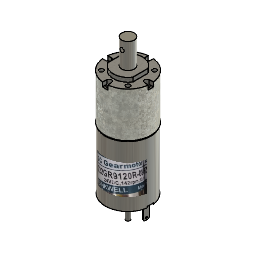
Hennkwell-PZ22GR9120R-084BBH-DC-gearmotor (Autodesk Fusion 360 design; units mm, degrees)
Autodesk Fusion 360 part; units mm, degrees
note: some values were not read from the file. Set by a fixed rule: which sketch regions a step uses.
sketch "Sketch1" plane through (0, 0, 0) normal (0, 1, 0) x (1, 0, 0)
  circle A0 centre (0, 0) radius 11
  circle A1 centre (0, 0) radius 10.8
  dimension "d1" = 22
  dimension "d4" = 21.6
  constraint coincident A0.centre A1.centre
  measures "d1" diameter of A0
  measures "d4" diameter of A1
extrude "Extrude1" add sketch "Sketch1" along normal blind 21.4 contours A0 | A1 makes body 1
extrude "Extrude2" add sketch "Sketch1" against normal blind 29.5 separate body contours A1 makes body 2
sketch "Sketch2" plane through (0, -29.5, 0) normal (0, -1, 0) x (1, 0, 0)
  circle A0 centre (0, 0) radius 10.8
  circle A1 centre (0, 0) radius 3.75
  circle A2 centre (0, 0) radius 1
  dimension "d7" = 7.5
  dimension "d8" = 2
  constraint concentric A0 A1
  constraint coincident A0.centre A1.centre
  measures "d7" diameter of A1
  measures "d8" diameter of A2
extrude "Extrude3" add sketch "Sketch2" along normal blind 2.5 contours A1 | A2 bodies 2
sketch "Sketch3" plane through (0, -29.5, 0) normal (0, -1, 0) x (1, 0, 0)
  circle A0 centre (0, 0) radius 3.75
  circle A1 centre (0, 0) radius 10.8
  line L0 (0, 0) -> (10.8, 0) construction
  line L1 (0, 0) -> (0, 10.8) construction
  line L2 (8.5, -1.5) -> (8.8, -1.5)
  line L3 (8.8, -1.5) -> (8.8, 1.5)
  line L4 (8.8, 1.5) -> (8.5, 1.5)
  line L5 (8.5, 1.5) -> (8.5, -1.5)
  line L6 (8.5, -1.5) -> (8.8, 1.5) construction
  line L7 (8.8, -1.5) -> (8.5, 1.5) construction
  line L8 (-8.8, -1.5) -> (-8.5, 1.5) construction
  line L9 (-8.5, 1.5) -> (-8.5, -1.5)
  line L10 (-8.8, -1.5) -> (-8.8, 1.5)
  line L11 (0, 0) -> (-10.8, 0) construction
  line L12 (-8.5, -1.5) -> (-8.8, 1.5) construction
  line L13 (-8.8, 1.5) -> (-8.5, 1.5)
  line L14 (-8.5, -1.5) -> (-8.8, -1.5)
  line L15 (-8.8, 1.5) -> (-10.6953, 1.5)
  line L16 (-8.8, -1.5) -> (-10.6953, -1.5)
  circle A2 centre (0, 0) radius 10.8
  line L17 (8.8, 1.5) -> (10.6953, 1.5)
  line L18 (8.8, -1.5) -> (10.6953, -1.5)
  point P0 (8.65, 0)
  dimension "d14" = 0.3
  dimension "d15" = 3
  dimension "d16" = 2
  constraint coincident A0.centre A1.centre
  constraint coincident A1 L0.end
  constraint horizontal L0
  constraint coincident A1 L1.end
  constraint perpendicular L0 L1
  constraint horizontal L2
  constraint perpendicular L2 L3
  constraint parallel L2 L4
  constraint parallel L3 L5
  constraint coincident L6 P0
  constraint coincident L7 P0
  constraint coincident L0 P0
  constraint symmetric A0.centre L1 A1.centre
  constraint symmetric L0.end L1 L11.end
  constraint symmetric L1 L2.start L9.end
  constraint symmetric L1 L2.end L8.start
  constraint symmetric L1 L3.end L10.end
  constraint symmetric L1 L4.end L8.end
  constraint coincident A1 L15.end
  constraint perpendicular L10 L15
  constraint coincident A1 L16.end
  constraint perpendicular L10 L16
  constraint coincident A2 L17.end
  constraint perpendicular L3 L17
  constraint coincident A2 L18.end
  constraint perpendicular L3 L18
  measures "d14" distance of L3.end L4.end
  measures "d15" distance of L2.end L3.end
  measures "d16" distance of L0.end L3
extrude "Extrude5" add sketch "Sketch3" along normal blind 6.75 contours L2 L3 L4 L5 | L9 L10 L13 L14 bodies 2
sketch "Sketch4" plane through (-8.8, 0, 0) normal (-1, 0, 0) x (0, 0, 1)
  line L0 (1.5, -29.5) -> (-1.5, -29.5)
  line L1 (-1.5, -29.5) -> (-1.5, -36.25)
  line L2 (-1.5, -36.25) -> (1.5, -36.25)
  line L3 (1.5, -36.25) -> (1.5, -29.5)
  circle A0 centre (0, -35.25) radius 0.5
  dimension "d19" = 1
  dimension "d20" = 1
  dimension "d21" = 1.5
  measures "d19" diameter of A0
  measures "d20" distance of L2 A0.centre
  measures "d21" distance of L1 A0.centre
extrude "Extrude6" cut sketch "Sketch4" against normal blind 1000 contours A0 bodies 2
fillet "Fillet1" radius 1 4 edges at (-8.65, -36.25, -1.5) (-8.65, -36.25, 1.5) (8.65, -36.25, 1.5) (8.65, -36.25, -1.5) on bodies 2
extrude "Extrude7" add sketch "Sketch2" along normal blind 8.4 from surface at 2.5 separate body contours A2 makes body 3
sketch "Sketch5" plane through (0, 21.4, 0) normal (0, 1, 0) x (-1, 0, 0)
  circle A0 centre (0, 0) radius 11
  line L0 (6, -3.625) -> (-6, -3.625)
  line L1 (-6, -3.625) -> (-6, 3.625)
  line L2 (-6, 3.625) -> (6, 3.625)
  line L3 (6, 3.625) -> (6, -3.625)
  line L4 (6, -3.625) -> (-6, 3.625) construction
  line L5 (-6, -3.625) -> (6, 3.625) construction
  line L6 (6, -3.625) -> (6, 3.625)
  arc A1 (-6, -3.6056) -> (6, -3.6056) centre (0, 0) ccw
  arc A2 (6, 3.6056) -> (-6, 3.6056) centre (0, 0) ccw
  circle A3 centre (0, 0) radius 3
  circle A4 centre (0, 0) radius 9
  line L7 (0, 0) -> (0, -11) construction
  line L8 (0, 0) -> (0, 11) construction
  line L9 (0, 0) -> (-11, 0) construction
  line L10 (0, 0) -> (11, 0) construction
  circle A5 centre (9, 0) radius 1.15
  circle A6 centre (0, 9) radius 1.15
  circle A7 centre (-9, 0) radius 1.15
  circle A8 centre (0, -9) radius 1.15
  line L11 (8.9265, -1.1477) -> (10.9258, -1.2756)
  line L12 (8.9265, 1.1477) -> (10.9258, 1.2756)
  line L13 (-8.9265, -1.1477) -> (-10.9258, -1.2756)
  line L14 (-8.9265, 1.1477) -> (-10.9258, 1.2756)
  line L15 (-1.1477, -8.9265) -> (-1.2756, -10.9258)
  line L16 (1.1477, -8.9265) -> (1.2756, -10.9258)
  line L17 (1.1477, 8.9265) -> (1.2756, 10.9258)
  line L18 (-1.1477, 8.9265) -> (-1.2756, 10.9258)
  line L19 (0, 0) -> (-6.3679, 6.36) construction
  circle A9 centre (-6.3679, 6.36) radius 1
  circle A10 centre (6.3679, 6.36) radius 1
  circle A11 centre (-6.3679, -6.36) radius 1
  circle A12 centre (6.3679, -6.36) radius 1
  dimension "d32" = 14
  dimension "d33" = 12
  dimension "d34" = 7.25
  dimension "d37" = 6
  dimension "d40" = 18
  dimension "d41" = 2.3
  dimension "d42" = 2.3
  dimension "d43" = 2.3
  dimension "d44" = 2.3
  dimension "d49" = 2
  constraint coincident A0.centre A1.centre
  constraint horizontal L0
  constraint perpendicular L0 L1
  constraint parallel L0 L2
  constraint parallel L1 L3
  constraint coincident L4 A0.centre
  constraint coincident L5 A0.centre
  constraint coincident L1 A2.end
  constraint coincident L1 A1.start
  constraint coincident L3 A1.end
  constraint coincident L3 A2.start
  constraint concentric A1 A2
  constraint concentric A1 A4
  constraint coincident A0 L7.end
  constraint perpendicular L0 L7
  constraint coincident A0 L8.end
  constraint parallel L7 L8
  constraint coincident A0 L9.end
  constraint perpendicular L8 L9
  constraint coincident A0 L10.end
  constraint perpendicular L3 L10
  constraint coincident A4 A5.centre
  constraint coincident L10 A5.centre
  constraint coincident A4 A6.centre
  constraint coincident L8 A6.centre
  constraint coincident A4 A7.centre
  constraint coincident L9 A7.centre
  constraint coincident A4 A8.centre
  constraint coincident L7 A8.centre
  constraint coincident A5 L11.start
  constraint coincident A4 L11.start
  constraint coincident A0 L11.end
  constraint tangent A5 L11
  constraint symmetric L10 L11.start L12.start
  constraint symmetric L10 L11.end L12.end
  constraint symmetric L8 L11.start L13.start
  constraint symmetric L8 L11.end L13.end
  constraint symmetric L8 L12.start L14.start
  constraint symmetric L8 L12.end L14.end
  constraint coincident A8 L15.start
  constraint coincident A4 L15.start
  constraint coincident A0 L15.end
  constraint tangent A8 L15
  constraint symmetric L7 L15.start L16.start
  constraint symmetric L7 L15.end L16.end
  constraint symmetric L10 L15.start L18.start
  constraint symmetric L10 L15.end L18.end
  constraint symmetric L10 L16.start L17.start
  constraint symmetric L10 L16.end L17.end
  constraint coincident A4 L19.end
  constraint coincident L19.end A9.centre
  constraint symmetric L8 A9 A10
  constraint symmetric L10 A9 A11
  constraint symmetric L10 A10 A12
  measures "d32" diameter of A1
  measures "d33" distance of L1.end L2.end
  measures "d34" distance of L0.end L1.end
  measures "d37" diameter of A3
  measures "d40" diameter of A4
  measures "d41" diameter of A5
  measures "d42" diameter of A6
  measures "d43" diameter of A7
  measures "d44" diameter of A8
  measures "d49" diameter of A9
extrude "Extrude8" add sketch "Sketch5" along normal blind 2 contours L0 A1 | L0 L1 L2 L3 L6 A1 A2 | L2 A2 | A3 bodies 1
extrude "Extrude9" add sketch "Sketch5" along normal blind 14 contours A3 bodies 1
extrude "Extrude10" cut sketch "Sketch5" against normal blind 2 contours A0 A5 L11 L12 | A0 A6 L17 L18 | A4 A5 | A4 A5 | A0 A8 L15 L16 | A4 A6 | A4 A6 | A4 A8 | A4 A8 | A0 A7 L13 L14 | A4 A7 | A4 A7 bodies 1
extrude "Extrude11" cut sketch "Sketch5" against normal blind 6.5 contours A4 A5 | A4 A5 | A4 A6 | A4 A6 | A4 A8 | A4 A8 | A4 A7 | A4 A7 bodies 1
extrude "Extrude12" cut sketch "Sketch5" against normal blind 4 contours A4 A10 | A4 A10 | A4 A12 | A4 A12 | A4 A9 | A4 A9 | A4 A11 | A4 A11 bodies 1
ref_plane "WorkPlane1" through (0, 31.7967, 3) normal (0, 0, 1) x (-1, 0, 0)
sketch "Sketch6" plane through (0, 0, 3) normal (0, 0, 1) x (1, 0, 0)
  line L0 (3, 35.4) -> (-3, 35.4)
  line L1 (-3, 23.4) -> (3, 23.4)
  circle A0 centre (0, 31.3) radius 1
  dimension "d53" = 2
  dimension "d54" = 4.1
  measures "d53" diameter of A0
  measures "d54" distance of L0 A0.centre
extrude "Extrude13" cut sketch "Sketch6" against normal blind 99 bodies 1
fillet "Fillet2" radius 0.5 1 edges at (-10.0691, 0, 3.9054) on bodies 2
extrude "Extrude14" cut sketch "Sketch3" against normal blind 0.6 contours A1 L3 A2 L17 L18 | A1 L10 L15 L16 A2 bodies 2
combine "Combine1" operation add target body 2 tool bodies 3
combine "Combine2" operation add target body 1 tool bodies 2
